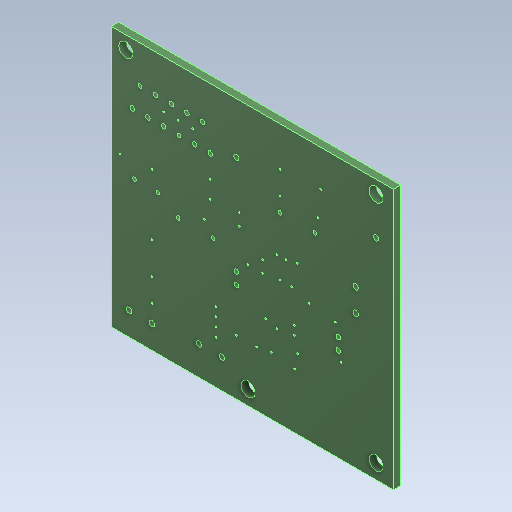
# Autodesk Inventor part: MPS_Drive_Amp_2.brd_Outline
Saved by Autodesk Inventor 2021 (Build 250183000, 183)
## iProperties
Created: 2020-11-18
Part Number: MPS_Drive_Amp_2.brd_Outline
Material: Generic
Document SubType Name: Modeling
Designer: Admin
Density: 1 g/cm^3
Appearance: Board Outline
Author: Admin
Autodesk Inventor part; units mm, degrees
ref_plane "YZ Plane" through (0, 0, 0) normal (1, 0, 0) x (0, 1, 0)
ref_plane "XZ Plane" through (0, 0, 0) normal (0, 1, 0) x (-1, 0, 0)
ref_plane "XY Plane" through (0, 0, 0) normal (0, 0, 1) x (1, 0, 0)
sketch "Sketch1" plane through (0, 0, 0) normal (0, 0, 1) x (1, 0, 0)
  line L0 (0, 0) -> (61.575, 0)
  line L1 (61.575, 0) -> (61.575, 56.82)
  line L2 (61.575, 56.82) -> (0, 56.82)
  line L3 (0, 56.82) -> (0, 0)
  circle A0 centre (10.16, 30.48) radius 0.405
  circle A1 centre (5.08, 30.48) radius 0.405
  circle A2 centre (22.23, 27.94) radius 0.405
  circle A3 centre (14.61, 27.94) radius 0.405
  circle A4 centre (44.45, 40.01) radius 0.405
  circle A5 centre (36.83, 40.01) radius 0.405
  circle A6 centre (27.3, 24.13) radius 0.51
  circle A7 centre (27.3, 21.59) radius 0.51
  circle A8 centre (49.53, 22.86) radius 0.51
  circle A9 centre (49.53, 20.32) radius 0.51
  circle A10 centre (27.3, 45.72) radius 0.55
  circle A11 centre (57.79, 45.72) radius 0.55
  circle A12 centre (4.57, 43.61) radius 0.5
  circle A13 centre (6.27, 48.69) radius 0.43
  circle A14 centre (7.98, 43.61) radius 0.5
  circle A15 centre (9.68, 48.69) radius 0.5
  circle A16 centre (11.38, 43.61) radius 0.5
  circle A17 centre (13.08, 48.69) radius 0.5
  circle A18 centre (14.78, 43.61) radius 0.43
  circle A19 centre (16.48, 48.69) radius 0.5
  circle A20 centre (18.19, 43.61) radius 0.5
  circle A21 centre (19.89, 48.69) radius 0.5
  circle A22 centre (21.59, 43.61) radius 0.5
  circle A23 centre (19.09, 6.35) radius 0.595
  circle A24 centre (24.09, 6.35) radius 0.595
  circle A25 centre (3.85, 5.08) radius 0.595
  circle A26 centre (8.85, 5.08) radius 0.595
  circle A27 centre (53.34, 34.25) radius 0.595
  circle A28 centre (53.34, 29.25) radius 0.595
  circle A29 centre (57.785, 3.175) radius 1.524
  circle A30 centre (3.175, 53.975) radius 1.524
  circle A31 centre (57.785, 53.975) radius 1.524
  circle A32 centre (29.845, 3.175) radius 1.524
  circle A33 centre (36.83, 27.305) radius 0.175
  circle A34 centre (39.37, 27.305) radius 0.175
  circle A35 centre (40.64, 32.385) radius 0.175
  circle A36 centre (20.32, 30.48) radius 0.175
  circle A37 centre (27.94, 33.02) radius 0.175
  circle A38 centre (27.94, 35.56) radius 0.175
  circle A39 centre (21.59, 34.925) radius 0.175
  circle A40 centre (21.59, 38.735) radius 0.175
  circle A41 centre (36.83, 43.18) radius 0.175
  circle A42 centre (45.085, 43.18) radius 0.175
  circle A43 centre (36.83, 48.26) radius 0.175
  circle A44 centre (45.72, 48.895) radius 0.175
  circle A45 centre (40.005, 20.32) radius 0.175
  circle A46 centre (40.005, 18.415) radius 0.175
  circle A47 centre (40.005, 12.065) radius 0.175
  circle A48 centre (31.75, 12.065) radius 0.175
  circle A49 centre (27.305, 12.065) radius 0.175
  circle A50 centre (8.89, 8.89) radius 0.175
  circle A51 centre (8.89, 13.97) radius 0.175
  circle A52 centre (8.89, 20.955) radius 0.175
  circle A53 centre (8.89, 34.29) radius 0.175
  circle A54 centre (1.905, 33.655) radius 0.175
  circle A55 centre (11.43, 46.355) radius 0.175
  circle A56 centre (14.605, 46.355) radius 0.175
  circle A57 centre (43.18, 26.035) radius 0.175
  circle A58 centre (50.165, 18.415) radius 0.175
  circle A59 centre (48.895, 25.4) radius 0.175
  circle A60 centre (33.655, 18.415) radius 0.175
  circle A61 centre (17.78, 46.355) radius 0.175
  circle A62 centre (33.02, 26.67) radius 0.175
  circle A63 centre (29.845, 26.67) radius 0.175
  circle A64 centre (33.02, 29.21) radius 0.175
  circle A65 centre (22.86, 9.525) radius 0.175
  circle A66 centre (22.86, 11.43) radius 0.175
  circle A67 centre (22.86, 13.335) radius 0.175
  circle A68 centre (22.86, 15.24) radius 0.175
  circle A69 centre (36.195, 31.75) radius 0.175
  circle A70 centre (34.925, 12.7) radius 0.175
  circle A71 centre (38.1, 31.75) radius 0.175
  circle A72 centre (40.64, 15.24) radius 0.175
  circle A73 centre (36.195, 17.78) radius 0.175
  constraints: 74 centre point, 8 end point
extrude "MPS_Drive_Amp_2.brd_Outline" add sketch "Sketch1" along normal blind 1.6
body "Solid1"
